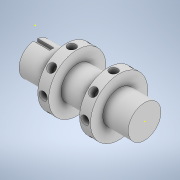
# Autodesk Inventor part: Shaft
Saved by Autodesk Inventor 2022 (Build 260153000, 153)
## iProperties
Created: 2021-10-30
Part Number: Shaft
Material: Generic
Document SubType Name: Modeling
Designer: raymo
Density: 1 g/cm^3
Appearance: Default
Author: raymo
Autodesk Inventor part; units mm, degrees
ref_plane "YZ Plane" through (0, 0, 0) normal (1, 0, 0) x (0, 1, 0)
sketch "Sketch1" plane through (0, 0, 0) normal (1, 0, 0) x (0, 1, 0)
  circle A0 centre (0, 0) radius 38.1
  dimension "d0" = 76.2
  constraints: 1 centre point, 1 coincident
  measures "d0" diameter of A0
extrude "Extrusion1" add sketch "Sketch1" along normal blind 254
sketch "Sketch2" plane through (0, 0, 0) normal (-1, 0, 0) x (0, 0, 1)
  line L0 (-5.08, 31.0851) -> (-5.08, 37.7598)
  circle A0 centre (0, 0) radius 38.1 projected
  line L1 (5.08, 31.0851) -> (5.08, 37.7598)
  line L2 (-5.08, 31.0851) -> (5.08, 31.0851)
  arc A1 (5.08, 37.7598) -> (-5.08, 37.7598) centre (0, 0) ccw
  constraints: 6 end point, 2 point on circle, 1 centre point, 1 perpendicular, 1 vertical, 3 other
extrude "Extrusion2" cut sketch "Sketch2" against normal blind 38.1 contours L0 A0 L1 L2 picked at (0.5659, 33.4108)
ref_plane "Work Plane1" through (169.418, 0, 0) normal (1, 0, 0) x (0, 0, -1)
ref_plane "Work Plane2" through (84.836, 0, 0) normal (1, 0, 0) x (0, 0, -1)
sketch "Sketch3" plane through (169.418, 0, 0) normal (1, 0, 0) x (0, 0, -1)
  circle A0 centre (0, 0) radius 66.675
  dimension "d9" = 133.35
  constraints: 1 centre point, 1 coincident
  measures "d9" diameter of A0
extrude "Extrusion3" add sketch "Sketch3" along normal blind 25.4
sketch "Sketch4" plane through (84.836, 0, 0) normal (1, 0, 0) x (0, 0, -1)
  point P0 (0, 0)
sketch "Sketch5" plane through (84.836, 0, 0) normal (1, 0, 0) x (0, 0, -1)
  circle A0 centre (0, 0) radius 66.675
  dimension "d12" = 133.35
  constraints: 1 centre point, 1 coincident
  measures "d12" diameter of A0
extrude "Extrusion4" add sketch "Sketch5" along normal mid plane 25.4
ref_plane "Work Plane3" through (169.418, 66.675, 0) normal (0, 1, 0) x (1, 0, 0)
sketch "Sketch6" plane through (169.418, 66.675, 0) normal (0, 1, 0) x (1, 0, 0)
  circle A0 centre (12.7, 0) radius 9.525
  circle A1 centre (-84.582, 0) radius 9.525
  point P0 (-169.418, 0)
  dimension "d15" = 19.05
  dimension "d16" = 19.05
  constraints: 2 centre point
  measures "d15" diameter of A0
  measures "d16" diameter of A1
extrude "Extrusion5" cut sketch "Sketch6" against normal blind 19.05
sketch "Sketch7" plane through (254, 0, 0) normal (1, 0, 0) x (0, 0, -1)
  point P0 (0, 0)
ref_plane "Work Plane4" through (0, 0, 66.675) normal (0, 0, 1) x (1, 0, 0)
sketch "Sketch8" plane through (0, 0, 66.675) normal (0, 0, 1) x (1, 0, 0)
  circle A0 centre (182.118, 0) radius 9.525
  circle A1 centre (84.836, 0) radius 9.525
  point P0 (0, 0)
  dimension "d20" = 19.05
  dimension "d21" = 19.05
  constraints: 2 centre point
  measures "d20" diameter of A0
  measures "d21" diameter of A1
sketch "Sketch9" plane through (84.836, 0, 0) normal (1, 0, 0) x (0, 0, -1)
  point P0 (0, 0)
sketch "Sketch10" plane through (169.418, 66.675, 0) normal (0, 1, 0) x (1, 0, 0)
  point P0 (-169.418, 0)
extrude "Extrusion6" cut sketch "Sketch8" against normal blind 19.05
ref_plane "Work Plane5" through (169.418, -66.675, 0) normal (0, 1, 0) x (1, 0, 0)
ref_plane "Work Plane6" through (0, 0, -66.675) normal (0, 0, 1) x (1, 0, 0)
sketch "Sketch11" plane through (169.418, -66.675, 0) normal (0, 1, 0) x (1, 0, 0)
  circle A0 centre (12.7, 0) radius 9.525
  circle A1 centre (-84.582, 0) radius 9.525 projected
  circle A2 centre (-84.582, 0) radius 9.525
  point P0 (-169.418, 0)
  dimension "d26" = 19.05
  constraints: 2 centre point, 1 coincident
  measures "d26" diameter of A0
extrude "Extrusion7" cut sketch "Sketch11" along normal blind 19.05
sketch "Sketch12" plane through (0, 0, -66.675) normal (0, 0, 1) x (1, 0, 0)
  circle A0 centre (84.836, 0) radius 9.525
  circle A1 centre (182.118, 0) radius 9.525 projected
  circle A2 centre (182.118, 0) radius 9.525
  point P0 (0, 0)
  constraints: 2 centre point, 1 coincident
extrude "Extrusion8" cut sketch "Sketch12" along normal blind 19.05
ref_plane "Work Plane7" through (169.418, 0, 66.675) normal (0, 0, 1) x (1, 0, 0)
pattern_circular "Circular Pattern1" count 8 over 360 about axis through (0, 0, 0) along (1, 0, 0) of "Extrusion8"
body "Solid1"
